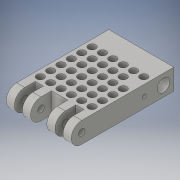
# Autodesk Inventor part: right wing
Saved by Autodesk Inventor 2016 SP2 (Build 200236200, 236)
## iProperties
Created: 2016-11-23
Part Number: right wing
Material: Aluminum 6061
Document SubType Name: Modeling
Designer: Teta
Density: 2.7 g/cm^3
Appearance: Aluminum - Flat
Author: Teta
Autodesk Inventor part; units mm, degrees
ref_plane "YZ Plane" through (0, 0, 0) normal (1, 0, 0) x (0, 1, 0)
ref_plane "XZ Plane" through (0, 0, 0) normal (0, 1, 0) x (-1, 0, 0)
ref_plane "XY Plane" through (0, 0, 0) normal (0, 0, 1) x (1, 0, 0)
sketch "Sketch1" plane through (0, 0, 0) normal (0, 1, 0) x (-1, 0, 0)
  line L0 (0, 0) -> (30.1498, 0)
  line L1 (30.1498, 0) -> (30.1498, -30.1498)
  line L2 (30.1498, -30.1498) -> (0, -30.1498)
  line L3 (0, -30.1498) -> (0, 0)
  dimension "d0" = 30.1498
  dimension "d1" = 30.1498
  constraints: 8 end point, 2 parallel, 1 horizontal, 1 perpendicular
  measures "d0" distance of L1.end L2.end
  measures "d1" distance of L0.end L1.end
extrude "Extrusion1" add sketch "Sketch1" along normal blind 9.652
sketch "Sketch3" plane through (0, 9.652, 0) normal (0, 1, 0) x (1, 0, 0)
  line L0 (-30.1498, 0) -> (0, 0) projected
  line L1 (0, 0) -> (0, 30.1498) projected
  line L2 (0, 30.1498) -> (-30.1498, 30.1498) projected
  line L3 (-30.1498, 30.1498) -> (-30.1498, 0) projected
  line L4 (-30.1498, 0) -> (0, 0) projected
  line L5 (-15.0749, 0) -> (-28.7909, 0)
  line L6 (-30.1498, 30.1498) -> (-30.1498, 0) projected
  line L7 (-30.1498, 15.0749) -> (-30.1498, 1.3589)
  line L8 (-30.1498, 1.3589) -> (-30.1498, 3.0861)
  line L9 (-30.1498, 3.0861) -> (-27.0637, 3.0861)
  line L10 (-28.7909, 0) -> (-27.0637, 0)
  line L11 (-27.0637, 0) -> (-27.0637, 3.0861)
  circle A0 centre (-27.0637, 3.0861) radius 1.7272
  line L12 (-15.0749, 0) -> (-15.0749, 4.3585)
  line L13 (-30.1498, 15.0749) -> (-29.1171, 15.0749)
  circle A1 centre (-3.0861, 3.0861) radius 1.7272
  line L14 (0, 15.0749) -> (-1.0327, 15.0749)
  circle A2 centre (-27.0637, 27.0637) radius 1.7272
  circle A3 centre (-3.0861, 27.0637) radius 1.7272
  dimension "d9" = 13.716
  dimension "d10" = 13.716
  dimension "d11" = 1.7272
  dimension "d12" = 1.7272
  dimension "d13" = 3.4544
  constraints: 18 end point, 5 symmetric about line, 4 centre point, 4 point on line, 2 midpoint, 2 perpendicular, 1 coincident, 1 horizontal, 1 vertical, 3 other
  measures "d9" distance of L5.start L5.end
  measures "d10" distance of L7.start L7.end
  measures "d11" distance of L7.end L8.end
  measures "d12" distance of L5.end L10.end
  measures "d13" diameter of A0
extrude "Extrusion3" cut sketch "Sketch3" against normal blind 30.48 contours A0 L9 L11 | L11 L9 A0 | A1 | A2 | A3
sketch "Sketch4" plane through (0, 0, 0) normal (1, 0, 0) x (0, 0, -1)
  line L0 (4.8133, 9.652) -> (4.8133, 0) projected
  line L1 (1.3589, 9.652) -> (1.3589, 0) projected
  line L2 (4.8133, 4.826) -> (9.6393, 4.826)
  circle A0 centre (4.9912, 4.826) radius 2.921 projected
  line L3 (30.1498, 0) -> (0, 0) projected
  line L4 (30.1498, 0) -> (30.1498, 9.652) projected
  line L5 (0, 9.652) -> (30.1498, 9.652) projected
  line L6 (0, 0) -> (0, 9.652) projected
  line L7 (0, 4.826) -> (-2.921, 4.826)
  circle A1 centre (-2.921, 4.826) radius 2.921
  line L8 (0, 0) -> (-7.747, 0)
  line L9 (-7.747, 0) -> (-7.747, 9.652)
  line L10 (-7.747, 9.652) -> (0, 9.652)
  line L11 (0, 9.652) -> (0, 0)
  dimension "d16" = 4.826
  dimension "d18" = 2.921
  dimension "d19" = 7.747
  constraints: 12 end point, 3 horizontal, 2 midpoint, 2 parallel, 1 centre point, 1 coincident, 1 perpendicular
  measures "d16" distance of L2.start L2.end
  measures "d18" distance of L7.start L7.end
  measures "d19" distance of L9.end L10.end
extrude "Extrusion4" add sketch "Sketch4" against normal up to surface (30.1498 mm away) contours L6 L8 L9 L10
sketch "Sketch5" plane through (0, 9.652, 0) normal (0, 1, 0) x (1, 0, 0)
  circle A0 centre (-3.0861, 27.0637) radius 1.7272 projected
  circle A1 centre (-3.0861, 3.0861) radius 1.7272 projected
  circle A2 centre (-27.0637, 3.0861) radius 1.7272 projected
  circle A3 centre (-27.0637, 27.0637) radius 1.7272 projected
  line L0 (0, 30.1498) -> (0, -7.747) projected
  line L1 (0, 30.1498) -> (-30.1498, 30.1498) projected
  line L2 (-30.1498, 30.1498) -> (-30.1498, -7.747) projected
  line L3 (0, -7.747) -> (-30.1498, -7.747) projected
  circle A4 centre (-27.0637, 27.0637) radius 1.7272
  circle A5 centre (-27.0637, 22.2631) radius 1.7272
  circle A6 centre (-27.0637, 17.4625) radius 1.7272
  circle A7 centre (-27.0637, 12.6619) radius 1.7272
  circle A8 centre (-27.0637, 7.8613) radius 1.7272
  circle A9 centre (-27.0637, 3.0607) radius 1.7272
  circle A10 centre (-22.2631, 27.0637) radius 1.7272
  circle A11 centre (-22.2631, 22.2631) radius 1.7272
  circle A12 centre (-22.2631, 17.4625) radius 1.7272
  circle A13 centre (-22.2631, 12.6619) radius 1.7272
  circle A14 centre (-22.2631, 7.8613) radius 1.7272
  circle A15 centre (-22.2631, 3.0607) radius 1.7272
  circle A16 centre (-17.4625, 27.0637) radius 1.7272
  circle A17 centre (-17.4625, 22.2631) radius 1.7272
  circle A18 centre (-17.4625, 17.4625) radius 1.7272
  circle A19 centre (-17.4625, 12.6619) radius 1.7272
  circle A20 centre (-17.4625, 7.8613) radius 1.7272
  circle A21 centre (-17.4625, 3.0607) radius 1.7272
  circle A22 centre (-12.6619, 27.0637) radius 1.7272
  circle A23 centre (-12.6619, 22.2631) radius 1.7272
  circle A24 centre (-12.6619, 17.4625) radius 1.7272
  circle A25 centre (-12.6619, 12.6619) radius 1.7272
  circle A26 centre (-12.6619, 7.8613) radius 1.7272
  circle A27 centre (-12.6619, 3.0607) radius 1.7272
  circle A28 centre (-7.8613, 27.0637) radius 1.7272
  circle A29 centre (-7.8613, 22.2631) radius 1.7272
  circle A30 centre (-7.8613, 17.4625) radius 1.7272
  circle A31 centre (-7.8613, 12.6619) radius 1.7272
  circle A32 centre (-7.8613, 7.8613) radius 1.7272
  circle A33 centre (-7.8613, 3.0607) radius 1.7272
  circle A34 centre (-3.0607, 27.0637) radius 1.7272
  circle A35 centre (-3.0607, 22.2631) radius 1.7272
  circle A36 centre (-3.0607, 17.4625) radius 1.7272
  circle A37 centre (-3.0607, 12.6619) radius 1.7272
  circle A38 centre (-3.0607, 7.8613) radius 1.7272
  circle A39 centre (-3.0607, 3.0607) radius 1.7272
  point P0 (0, 0)
  dimension "d24" = 4.8006
  dimension "d27" = 4.8006
  constraints: 36 centre point, 1 coincident, 1 concentric, 1 horizontal, 1 vertical, 70 other
  measures "d24" distance of A4.centre A5.centre
  measures "d27" distance of A4.centre A10.centre
extrude "Extrusion5" cut sketch "Sketch5" against normal blind 30.48 contours A5 | A6 | A7 | A8 | A10 | A11 | A12 | A13 | A14 | A15 | A16 | A17 | A18 | A19 | A20 | A21 | A22 | A23 | A24 | A25 | A26 | A27 | A28 | A29 | A30 | A31 | A32 | A33 | A35 | A36 | A37 | A38
sketch "Sketch6" plane through (0, 0, -30.1498) normal (1, 0, 0) x (0, 0, -1)
  circle A0 centre (-33.0708, 4.826) radius 2.921 projected
  line L0 (0, 9.652) -> (-37.8968, 9.652) projected
  line L1 (-37.8968, 9.652) -> (-37.8968, 0) projected
  line L2 (-37.8968, 0) -> (0, 0) projected
  line L3 (0, 0) -> (0, 9.652) projected
  line L4 (-24.0157, 9.652) -> (-24.0157, 0) projected
  line L5 (-25.3365, 9.652) -> (-25.3365, 0) projected
  line L6 (-25.3365, 4.826) -> (-24.0157, 4.826)
  line L7 (-24.6761, 4.826) -> (-25.3365, 4.826)
  line L8 (-28.7909, 9.652) -> (-28.7909, 0) projected
  line L9 (-25.0063, 4.826) -> (-24.1173, 4.826)
  circle A1 centre (-24.1173, 4.826) radius 0.889
  point P0 (-30.1498, 0)
  dimension "d33" = 0.889
  dimension "d34" = 1.778
  constraints: 6 end point, 4 midpoint, 1 centre point, 1 coincident, 1 perpendicular, 1 point on line
  measures "d33" distance of L9.start L9.end
  measures "d34" diameter of A1
sketch "Sketch7" plane through (0, 9.652, 0) normal (0, 1, 0) x (1, 0, 0)
  circle A0 centre (-3.0607, 7.8613) radius 1.7272 projected
  point P0 (0, 0)
extrude "Extrusion6" add sketch "Sketch7" against normal blind 9.652
extrude "Extrusion7" cut sketch "Sketch6" against normal blind 6.35 contours A1 L4 | L4 L6 A1 | L4 A1 L6
sketch "Sketch8" plane through (0, 0, -30.1498) normal (1, 0, 0) x (0, 0, -1)
  circle A0 centre (-24.1173, 4.826) radius 0.889 projected
  circle A1 centre (-33.0708, 4.826) radius 2.921 projected
  line L0 (0, 9.652) -> (-37.8968, 9.652) projected
  line L1 (-37.8968, 9.652) -> (-37.8968, 0) projected
  line L2 (-37.8968, 0) -> (0, 0) projected
  line L3 (0, 0) -> (0, 9.652) projected
  line L4 (0, 0) -> (0, 9.652) projected
  line L5 (0, 4.826) -> (0, 0)
  line L6 (-1.3589, 0) -> (-4.8133, 0) projected
  line L7 (0, 4.826) -> (4.826, 4.826)
  circle A2 centre (4.826, 4.826) radius 4.826
  line L8 (0, 9.652) -> (4.826, 9.652)
  line L9 (4.826, 0) -> (0, 0)
  point P0 (-30.1498, 0)
  dimension "d39" = 4.826
  dimension "d40" = 4.826
  constraints: 8 end point, 2 horizontal, 2 point on circle, 1 centre point, 1 coincident, 1 midpoint, 1 parallel, 1 perpendicular
  measures "d39" distance of L5.start L2.end
  measures "d40" distance of L5.start L7.end
extrude "Extrusion8" add sketch "Sketch8" against normal up to surface (30.1498 mm away) contours L8 A2 L3 | A2 L9 L3 | A2
sketch "Sketch9" plane through (0, 0, 7.747) normal (1, 0, 0) x (0, 0, -1)
  circle A0 centre (13.7795, 4.826) radius 0.889 projected
  circle A1 centre (4.826, 4.826) radius 2.921 projected
  line L0 (42.7228, 9.652) -> (0, 9.652) projected
  line L1 (0, 9.652) -> (0, 0) projected
  line L2 (0, 0) -> (42.7228, 0) projected
  arc A2 (42.7228, 0) -> (42.7228, 9.652) centre (42.7228, 4.826) ccw projected
  circle A3 centre (42.7228, 4.826) radius 1.4986
  point P0 (7.747, 0)
  dimension "d43" = 2.9972
  constraints: 1 centre point, 1 coincident
  measures "d43" diameter of A3
extrude "Extrusion9" cut sketch "Sketch9" against normal through all contours A3
sketch "Sketch10" plane through (0, 9.652, 0) normal (0, 1, 0) x (1, 0, 0)
  circle A0 centre (-3.0607, 12.6619) radius 1.7272 projected
  circle A1 centre (-3.0607, 22.2631) radius 1.7272 projected
  circle A2 centre (-7.8613, 7.8613) radius 1.7272 projected
  circle A3 centre (-7.8613, 17.4625) radius 1.7272 projected
  circle A4 centre (-7.8613, 27.0637) radius 1.7272 projected
  circle A5 centre (-12.6619, 7.8613) radius 1.7272 projected
  circle A6 centre (-12.6619, 17.4625) radius 1.7272 projected
  circle A7 centre (-12.6619, 27.0637) radius 1.7272 projected
  circle A8 centre (-17.4625, 7.8613) radius 1.7272 projected
  circle A9 centre (-17.4625, 17.4625) radius 1.7272 projected
  circle A10 centre (-17.4625, 27.0637) radius 1.7272 projected
  circle A11 centre (-22.2631, 7.8613) radius 1.7272 projected
  circle A12 centre (-22.2631, 17.4625) radius 1.7272 projected
  circle A13 centre (-22.2631, 27.0637) radius 1.7272 projected
  circle A14 centre (-27.0637, 12.6619) radius 1.7272 projected
  circle A15 centre (-27.0637, 22.2631) radius 1.7272 projected
  circle A16 centre (-27.0637, 17.4625) radius 1.7272 projected
  circle A17 centre (-27.0637, 7.8613) radius 1.7272 projected
  circle A18 centre (-22.2631, 22.2631) radius 1.7272 projected
  circle A19 centre (-22.2631, 12.6619) radius 1.7272 projected
  circle A20 centre (-22.2631, 3.0607) radius 1.7272 projected
  circle A21 centre (-17.4625, 22.2631) radius 1.7272 projected
  circle A22 centre (-17.4625, 12.6619) radius 1.7272 projected
  circle A23 centre (-17.4625, 3.0607) radius 1.7272 projected
  circle A24 centre (-12.6619, 22.2631) radius 1.7272 projected
  circle A25 centre (-12.6619, 12.6619) radius 1.7272 projected
  circle A26 centre (-12.6619, 3.0607) radius 1.7272 projected
  circle A27 centre (-7.8613, 22.2631) radius 1.7272 projected
  circle A28 centre (-7.8613, 12.6619) radius 1.7272 projected
  circle A29 centre (-7.8613, 3.0607) radius 1.7272 projected
  circle A30 centre (-3.0607, 17.4625) radius 1.7272 projected
  circle A31 centre (-3.0861, 27.0637) radius 1.7272 projected
  circle A32 centre (-3.0861, 3.0861) radius 1.7272 projected
  circle A33 centre (-27.0637, 3.0861) radius 1.7272 projected
  circle A34 centre (-27.0637, 27.0637) radius 1.7272 projected
  line L0 (0, 34.9758) -> (0, -7.747) projected
  line L1 (0, 34.9758) -> (-30.1498, 34.9758) construction
  line L2 (-30.1498, 34.9758) -> (-30.1498, -7.747) projected
  line L3 (0, -7.747) -> (-30.1498, -7.747) projected
  line L4 (0, 36.4744) -> (-30.1498, 36.4744) construction
  line L5 (-30.1498, 34.9758) -> (-30.1498, 34.9758) projected
  line L6 (0, 34.9758) -> (-30.1498, 34.9758) construction
  line L7 (0, 34.9758) -> (0, 34.9758) projected
  line L8 (0, 34.9758) -> (-30.1498, 34.9758) projected
  line L9 (-30.1498, 34.9758) -> (-30.1498, 39.8018) projected
  line L10 (0, 34.9758) -> (0, 39.8018) projected
  line L11 (0, 33.4772) -> (-30.1498, 33.4772) construction
  line L12 (-30.1498, 34.9758) -> (-30.1498, -7.747) projected
  line L13 (-30.1498, 30.076) -> (0, 30.076)
  line L14 (0, 30.076) -> (0, 39.8018)
  line L15 (-30.1498, 39.8018) -> (-30.1498, 30.076)
  line L16 (-15.0749, 39.8018) -> (-15.0749, 30.076)
  line L17 (0, 34.9758) -> (-30.1498, 34.9758) projected
  line L18 (-15.0749, 34.9758) -> (-30.1498, 34.9758) construction
  line L19 (-30.1498, 34.9758) -> (-22.6123, 34.9758)
  line L20 (-22.6123, 34.9758) -> (-22.6123, 39.8018)
  line L21 (-22.6123, 34.9758) -> (-22.6123, 30.076)
  line L22 (0, 34.9758) -> (-7.5374, 34.9758)
  line L23 (-7.5374, 39.8018) -> (-7.5374, 30.076)
  line L24 (-26.3811, 30.076) -> (-26.3811, 39.8018)
  line L25 (-22.6123, 30.076) -> (-15.0749, 30.076)
  line L26 (-18.8436, 30.076) -> (-18.8436, 39.8018)
  line L27 (-7.5374, 30.076) -> (-15.0749, 30.076)
  line L28 (-11.3062, 30.076) -> (-11.3062, 39.8018)
  line L29 (0, 30.076) -> (-7.5374, 30.076)
  line L30 (-3.7687, 30.076) -> (-3.7687, 39.8018)
  line L31 (-3.7687, 30.076) -> (-7.5374, 30.076)
  line L32 (-7.5374, 30.076) -> (-7.5374, 39.8018)
  line L33 (-7.5374, 39.8018) -> (-3.7687, 39.8018)
  line L34 (-3.7687, 39.8018) -> (-3.7687, 30.076)
  line L35 (-11.3062, 30.076) -> (-15.0749, 30.076)
  line L36 (-15.0749, 30.076) -> (-15.0749, 39.8018)
  line L37 (-15.0749, 39.8018) -> (-11.3062, 39.8018)
  line L38 (-11.3062, 39.8018) -> (-11.3062, 30.076)
  line L39 (-18.8436, 30.076) -> (-22.6123, 30.076)
  line L40 (-22.6123, 30.076) -> (-22.6123, 39.8018)
  line L41 (-18.8436, 39.8018) -> (-18.8436, 30.076)
  line L42 (-22.6123, 30.076) -> (-26.3811, 30.076)
  line L43 (-26.3811, 30.076) -> (-26.3811, 39.8018)
  line L44 (-26.3811, 39.8018) -> (-22.6123, 39.8018)
  line L45 (-22.6123, 39.8018) -> (-22.6123, 30.076)
  line L46 (-3.7687, 30.076) -> (-7.5374, 30.076)
  line L47 (-7.5374, 30.076) -> (-7.5374, 39.8018)
  line L48 (-7.5374, 39.8018) -> (-3.7687, 39.8018)
  line L49 (-3.7687, 39.8018) -> (-3.7687, 30.076)
  line L50 (-11.3062, 30.076) -> (-18.8436, 30.076)
  line L51 (-18.8436, 30.076) -> (-18.8436, 39.8018)
  line L52 (-18.8436, 39.8018) -> (-11.3062, 39.8018)
  line L53 (-11.3062, 39.8018) -> (-11.3062, 30.076)
  point P0 (0, 0)
  constraints: 80 end point, 12 parallel, 11 perpendicular, 8 horizontal, 6 midpoint, 5 point on line, 2 collinear, 1 vertical
extrude "Extrusion10" cut sketch "Sketch10" against normal through all contours L30 L13 L23 L8 | L8 L23 L33 L30 | L28 L13 L16 L8 | L8 L16 L37 L28 | L16 L13 L26 L8 | L8 L26 L52 L16 | L24 L8 L21 L13 | L24 L44 L20 L8
ref_plane "Work Plane1" through (0, 0, -43.053) normal (0, 0, 1) x (1, 0, 0)
mirror "Mirror1" about plane through (0, 0, -43.053) normal (0, 0, 1) remove original yes
body "Solid1"
